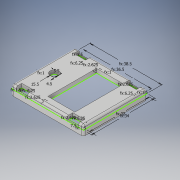
# Autodesk Inventor part: Lid
Saved by Autodesk Inventor 2019 (Build 230136000, 136)
## iProperties
Created: 2019-01-03
Part Number: Lid
Material: Generic
Document SubType Name: Sheet Metal
Designer: flato
Density: 1 g/cm^3
Appearance: Default
Sheet Metal Rule: Default
Author: flato
Autodesk Inventor part; units mm, degrees
ref_plane "YZ Plane" through (0, 0, 0) normal (1, 0, 0) x (0, 1, 0)
ref_plane "XZ Plane" through (0, 0, 0) normal (0, 1, 0) x (-1, 0, 0)
ref_plane "XY Plane" through (0, 0, 0) normal (0, 0, 1) x (1, 0, 0)
sketch "Sketch1" plane through (0, 0, 0) normal (0, 1, 0) x (-1, 0, 0)
  line L0 (7.978, 32.4505) -> (-28.522, 32.4505)
  line L1 (-28.522, 32.4505) -> (-28.522, 0.4505)
  line L2 (-28.522, 0.4505) -> (7.978, 0.4505)
  line L3 (7.978, 0.4505) -> (7.978, 32.4505)
  line L4 (8.978, 33.4505) -> (-29.522, 33.4505)
  line L5 (-29.522, 33.4505) -> (-29.522, -0.5495)
  line L6 (-29.522, -0.5495) -> (8.978, -0.5495)
  line L7 (8.978, -0.5495) -> (8.978, 33.4505)
  line L8 (-28.522, 32.4505) -> (-28.522, 33.4505)
  line L9 (7.978, 32.4505) -> (7.978, 33.4505)
  line L10 (7.978, 32.9505) -> (6.478, 32.9505)
  line L11 (7.978, 0.4505) -> (7.978, -0.5495)
  line L12 (-28.522, 0.4505) -> (-28.522, -0.5495)
  line L13 (-28.522, -0.0495) -> (-27.022, -0.0495)
  line L14 (6.478, 32.9505) -> (0.228, 32.9505)
  line L15 (0.228, 32.9505) -> (0.228, 30.3255)
  line L16 (0.228, 30.3255) -> (6.478, 30.3255)
  line L17 (6.478, 30.3255) -> (6.478, 32.9505)
  line L18 (6.478, -0.0495) -> (0.228, -0.0495)
  line L19 (0.228, -0.0495) -> (0.228, 2.5755)
  line L20 (0.228, 2.5755) -> (6.478, 2.5755)
  line L21 (6.478, 2.5755) -> (6.478, -0.0495)
  line L22 (-27.022, -0.0495) -> (-20.772, -0.0495)
  line L23 (-20.772, -0.0495) -> (-20.772, 2.5755)
  line L24 (-20.772, 2.5755) -> (-27.022, 2.5755)
  line L25 (-27.022, 2.5755) -> (-27.022, -0.0495)
  line L26 (-28.522, 32.9505) -> (-27.022, 32.9505)
  line L27 (-27.022, 32.9505) -> (-20.772, 32.9505)
  line L28 (-20.772, 32.9505) -> (-20.772, 30.3255)
  line L29 (-27.022, 30.3255) -> (-27.022, 32.9505)
  line L30 (-28.522, 0.4505) -> (-21.022, 0.4505)
  line L31 (-21.022, 32.4505) -> (-28.522, 32.4505)
  line L32 (-28.522, 32.4505) -> (-28.522, 0.4505)
  line L33 (-21.022, 3.4505) -> (-6.522, 3.4505)
  line L34 (-6.522, 3.4505) -> (-6.522, 0.4505)
  line L35 (-6.522, 3.4505) -> (-6.522, 29.4505)
  line L36 (-20.772, 30.3255) -> (-27.022, 30.3255)
  line L37 (6.478, -0.0495) -> (7.978, -0.0495)
  line L38 (-6.522, 29.4505) -> (-21.022, 29.4505)
  line L39 (-6.522, 29.4505) -> (-6.522, 32.4505)
  line L40 (-21.022, 3.4505) -> (-21.022, 29.4505)
  circle A0 centre (2.478, 16.9505) radius 2.25
  point P0 (0, 0)
  point P1 (-21.022, 31.4505)
  dimension "d0" = 36.5
  dimension "d1" = 32
  dimension "d4" = 38.5
  dimension "d5" = 34
  dimension "d6" = 1
  dimension "d7" = 1
  dimension "d31" = 1.5
  dimension "d33" = 1.5
  dimension "d34" = 6.25
  dimension "x1" = 6.25
  dimension "d36" = 6.25
  dimension "d37" = 2.625
  dimension "y1" = 2.625
  dimension "d39" = 2.625
  dimension "d42" = 1.5
  dimension "d44" = 2.625
  dimension "d69" = 7.5
  dimension "d82" = 3
  dimension "d84" = 6.25
  dimension "d85" = 1.5
  dimension "d88" = 3
  dimension "d89" = 4.5
  dimension "d90" = 15.5
  dimension "d91" = 5.5
  constraints: 82 end point, 13 parallel, 12 perpendicular, 11 horizontal, 8 point on line, 4 midpoint, 1 centre point, 1 vertical
  measures "d0" distance of L2.end L1.end
  measures "d1" distance of L0.end L1.end
  measures "d4" distance of L6.end L5.end
  measures "d5" distance of L4.end L5.end
  measures "d6" distance between parallel lines of L2 L6
  measures "d7" distance between parallel lines of L3 L7
  measures "d31" distance of L10.start L10.end
  measures "d33" distance of L13.start L13.end
  measures "d34" distance of L16.end L15.end
  measures "x1" distance of L19.end L20.end
  measures "d36" distance of L24.end L23.end
  measures "d37" distance of L22.end L23.end
  measures "y1" distance of L18.end L19.end
  measures "d39" distance of L14.end L15.end
  measures "d42" distance of L26.start L26.end
  measures "d44" distance of L27.end L28.end
  measures "d69" distance of L31.end L31.start
  measures "d82" distance of L33.end L34.end
  measures "d84" distance of L28.end L29.start
  measures "d85" distance of L18.start L37.end
  measures "d88" distance of L38.start L39.end
  measures "d89" diameter of A0
  measures "d90" distance from line of L0 A0.centre
  measures "d91" distance from line of L3 A0.centre
extrude "Extrusion1" add sketch "Sketch1" along normal blind 2.125 contours L9 L4 L7 L6 L11 L3 | L0 L17 L10 L9 | L0 L15 L14 L17 | L11 L37 L21 L2 | L10 L14 L15 L0 L28 L27 L26 L8 L4 L9 | L21 L18 L19 L2 | L11 L6 L12 L13 L22 L23 L2 L19 L18 L37 | L8 L1 L12 L6 L5 L4 | L0 L29 L27 L28 | L26 L29 L0 L8 | L23 L22 L25 L2 | L12 L2 L25 L13
fillet "Fillet1" radius 1 4 edges at (29.522, 1.0625, 33.4505) (29.522, 1.0625, -0.5495) (-8.978, 1.0625, -0.5495) (-8.978, 1.0625, 33.4505)
sketch "Sketch3" plane through (-7.978, 0, 0.4505) normal (0, 0, 1) x (1, 0, 0)
  point P0 (7.978, 0)
extrude "Extrusion2" add sketch "Sketch1" along normal blind 2.125 contours L3 L2 L21 L20 L19 L34 L35 L39 L0 L15 L16 L17 | L17 L16 L15 L0 | L2 L19 L20 L21 | L39 L38 L40 L33 L34 L2 L23 L24 L25 L1 L0 L29 L36 L28 | L28 L36 L29 L0 | L2 L25 L24 L23 | A0
extrude "Extrusion6" cut sketch "Sketch1" along normal blind 2.125 contours L28 L36 L29 L0 | L0 L29 L27 L28
extrude "Extrusion7" cut sketch "Sketch1" along normal blind 2.125 contours L17 L16 L15 L0 | L0 L15 L14 L17 | L21 L18 L19 L2 | L2 L19 L20 L21
extrude "Extrusion8" cut sketch "Sketch1" along normal blind 2.125 contours L23 L22 L25 L2 | L2 L25 L24 L23
sketch "Sketch11" plane through (0, 2.125, 0) normal (0, 1, 0) x (1, 0, 0)
  line L0 (-6.478, 0.0495) -> (-0.228, 0.0495) projected
  line L1 (28.522, 0.5495) -> (-7.978, 0.5495) projected
  line L2 (-6.478, 0.0495) -> (-0.228, 0.0495)
  line L3 (-0.228, 0.0495) -> (-0.228, 0.5495)
  line L4 (-0.228, 0.5495) -> (-6.478, 0.5495)
  line L5 (-6.478, 0.5495) -> (-6.478, 0.0495)
  line L6 (-6.478, -32.9505) -> (-6.478, -30.3255) projected
  line L7 (-7.978, -33.4505) -> (28.522, -33.4505) projected
  line L8 (-6.478, -32.9505) -> (-0.228, -32.9505)
  line L9 (-0.228, -32.9505) -> (-0.228, -33.4505)
  line L10 (-0.228, -33.4505) -> (-6.478, -33.4505)
  line L11 (-6.478, -33.4505) -> (-6.478, -32.9505)
  line L12 (27.022, -32.9505) -> (20.772, -32.9505) projected
  line L13 (20.772, -32.9505) -> (27.022, -32.9505)
  line L14 (27.022, -32.9505) -> (27.022, -33.4505)
  line L15 (27.022, -33.4505) -> (20.772, -33.4505)
  line L16 (20.772, -33.4505) -> (20.772, -32.9505)
  line L17 (20.772, 0.0495) -> (27.022, 0.0495) projected
  line L18 (20.772, 0.0495) -> (27.022, 0.0495)
  line L19 (27.022, 0.0495) -> (27.022, 0.5495)
  line L20 (27.022, 0.5495) -> (20.772, 0.5495)
  line L21 (20.772, 0.5495) -> (20.772, 0.0495)
  point P0 (0, 0)
  dimension "d55" = 6.25
  dimension "d56" = 6.25
  constraints: 32 end point, 8 parallel, 6 point on line, 4 horizontal, 4 perpendicular
  measures "d55" distance of L9.end L10.end
  measures "d56" distance of L14.end L15.end
extrude "Extrusion9" cut sketch "Sketch11" against normal blind 1.75
fillet "Fillet3" radius 1 12 edges at (-8.6851, 2.125, 33.1576) (-8.978, 2.125, 16.4505) (-8.6851, 2.125, -0.2566) (-7.228, 2.125, -0.5495) (10.272, 2.125, -0.5495) (27.772, 2.125, -0.5495) (27.772, 2.125, 33.4505) (10.272, 2.125, 33.4505) (-7.228, 2.125, 33.4505) (29.2291, 2.125, -0.2566) (29.2291, 2.125, 33.1576) (29.522, 2.125, 16.4505)
extrude "Extrusion16" add sketch "Sketch1" against normal blind 3 contours L9 L4 L7 L6 L11 L3 | L0 L17 L10 L9 | L0 L15 L14 L17 | L11 L37 L21 L2 | L10 L14 L15 L0 L28 L27 L26 L8 L4 L9 | L21 L18 L19 L2 | L11 L6 L12 L13 L22 L23 L2 L19 L18 L37 | L8 L1 L12 L6 L5 L4 | L0 L29 L27 L28 | L26 L29 L0 L8 | L23 L22 L25 L2 | L12 L2 L25 L13
fillet "Fillet5" radius 1 4 edges at (-8.978, -1.5, -0.5495) (-8.978, -1.5, 33.4505) (29.522, -1.5, 33.4505) (29.522, -1.5, -0.5495)
extrude "Extrusion17" cut sketch "Sketch1" against normal up to next contours L17 L16 L15 L0 | L0 L15 L14 L17 | L21 L18 L19 L2 | L2 L19 L20 L21 | L28 L36 L29 L0 | L0 L29 L27 L28 | L23 L22 L25 L2 | L2 L25 L24 L23
extrude "Extrusion18" cut sketch "Sketch1" along normal up to next contours A0
equation "\"d0\" = basey1"
equation "\"d1\" = basex1"
equation "\"d4\" = basey2"
equation "\"d5\" = basex2"
equation "\"d31\" = z1"
equation "\"d34\" = x1"
equation "\"d36\" = x1"
equation "\"d37\" = y1"
equation "\"d39\" = y1"
equation "\"d44\" = y1"
equation "\"d55\" = d34"
equation "\"d56\" = d43"
equation "\"d43\" = x1"
equation "\"basey1\" = 36.5"
equation "\"basex1\" = 32"
equation "\"basey2\" = 38.5"
equation "\"basex2\" = 34"
equation "\"z1\" = 1.5"
body "Solid1"
